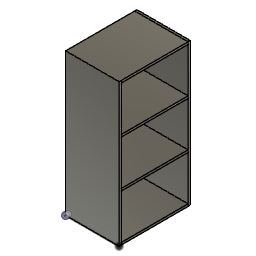
Shelf.3d v2 (Autodesk Fusion 360 design; units mm, degrees)
Autodesk Fusion 360 part; units mm, degrees
sketch "Sketch1" plane through (0, 0, 0) normal (0, 1, 0) x (1, 0, 0)
  line L0 (0, 0) -> (457.2, 0)
  line L1 (457.2, 0) -> (457.2, -1219.2)
  line L2 (457.2, -1219.2) -> (0, -1219.2)
  line L3 (0, -1219.2) -> (0, 0)
  dimension "d4" = 457.2
  dimension "d5" = 1219.2
  constraint horizontal L0
  constraint vertical L1
  constraint horizontal L2
  constraint vertical L3
  constraint coincident L0.start L3.end
  measures "d4" distance of L0.start L0.end
  measures "d5" distance of L0.start L2.end
extrude "Extrude1" add sketch "Sketch1" along normal blind 19.05 makes body 1
pattern_linear "R-Pattern1" count 2 spacing 590.55 along (0, 1, 0) of bodies 1 makes body 2
sketch "Sketch2" plane through (0, 0, 0) normal (0, 0, 1) x (1, 0, 0)
  line L0 (0, 0) -> (457.2, 0)
  line L1 (0, 0) -> (0, 19.05)
  dimension "d12" = 457.2
  dimension "d14" = 19.05
  constraint horizontal L0
  constraint coincident L0.start L1.start
  measures "d12" distance of L0.start L0.end
  measures "d14" distance of L0.start L1.end
sketch "Sketch3" plane through (0, 0, 0) normal (0, 0, 1) x (1, 0, 0)
sketch "Sketch4" plane through (0, 0, 0) normal (0, 0, 1) x (1, 0, 0)
  line L0 (457.2, 19.05) -> (0, 19.05)
  line L1 (0, 19.05) -> (0, 590.55)
  line L2 (0, 590.55) -> (457.2, 590.55)
  line L3 (457.2, 590.55) -> (457.2, 19.05)
  constraint horizontal L0
  constraint vertical L1
  constraint horizontal L2
  constraint vertical L3
extrude "Extrude2" add sketch "Sketch4" along normal blind 19.05 bodies 1
pattern_linear "R-Pattern2" count 4 spacing 400.05 along (0, 0, 1) of "Extrude2"
equation "shelfHeight = 48 in"
equation "ShelfDepths = 18 in"
equation "ShelfThickness = ( 3 / 4 ) * 1 in"
equation "d4 = ShelfDepths"
equation "d5 = shelfHeight"
equation "d6 = ShelfThickness"
equation "d10 = ShelfWidths - ShelfThickness"
equation "d12 = ShelfDepths"
equation "d14 = ShelfThickness"
equation "ShelfWidths = 24 in"
equation "d17 = ShelfThickness"
equation "d21 = -shelfHeight + ShelfThickness"
